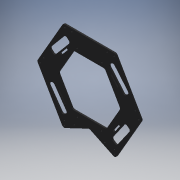
# Autodesk Inventor part: Bottom Plate
Saved by Autodesk Inventor 2017 (Build 210142000, 142)
## iProperties
Created: 2016-10-01
Part Number: Bottom Plate
Material: PVC, Unplasticized
Document SubType Name: Modeling
Designer: James Yelland
Density: 1.29 g/cm^3
Appearance: Smooth - White
Mass: 37.5584 g
Surface Area: 327.952 cm^2
Volume: 29.115 cm^3
Author: James Yelland
Autodesk Inventor part; units mm, degrees
ref_plane "YZ Plane" through (0, 0, 0) normal (1, 0, 0) x (0, 1, 0)
ref_plane "XZ Plane" through (0, 0, 0) normal (0, 1, 0) x (-1, 0, 0)
ref_plane "XY Plane" through (0, 0, 0) normal (0, 0, 1) x (1, 0, 0)
sketch "Sketch1" plane through (0, 0, 0) normal (0, 1, 0) x (-1, 0, 0)
  line L0 (68.7536, -48.1418) -> (56.7085, -65.344)
  line L1 (68.7536, -48.1418) -> (80.7987, -30.9396)
  line L2 (79.8164, -25.3687) -> (75.7207, -22.5008)
  line L3 (70.1498, -23.4831) -> (46.0595, -57.8875)
  line L4 (47.0418, -63.4584) -> (51.1376, -66.3263)
  arc A0 (51.1376, -66.3263) -> (56.7085, -65.344) centre (53.4319, -63.0497) ccw
  arc A1 (46.0595, -57.8875) -> (47.0418, -63.4584) centre (49.3361, -60.1818) ccw
  arc A2 (75.7207, -22.5008) -> (70.1498, -23.4831) centre (73.4264, -25.7774) ccw
  arc A3 (80.7987, -30.9396) -> (79.8164, -25.3687) centre (77.5221, -28.6453) ccw
  line L5 (-68.7536, -48.1418) -> (-80.7987, -30.9396)
  line L6 (-68.7536, -48.1418) -> (-56.7085, -65.344)
  line L7 (-51.1376, -66.3263) -> (-47.0418, -63.4584)
  line L8 (-46.0595, -57.8875) -> (-70.1496, -23.4833)
  line L9 (-75.7207, -22.5008) -> (-79.8164, -25.3687)
  arc A4 (-79.8164, -25.3687) -> (-80.7987, -30.9396) centre (-77.5221, -28.6453) ccw
  arc A5 (-70.1496, -23.4833) -> (-75.7207, -22.5008) centre (-73.4264, -25.7774) ccw
  arc A6 (-47.0418, -63.4584) -> (-46.0595, -57.8875) centre (-49.3361, -60.1818) ccw
  arc A7 (-56.7085, -65.344) -> (-51.1376, -66.3263) centre (-53.4319, -63.0497) ccw
  line L10 (103.5566, -2.5) -> (54.8095, -86.9325)
  line L11 (-54.8095, -86.9325) -> (-103.5566, -2.5)
  line L12 (-103.5566, 2.5) -> (-53.9434, 88.4327)
  line L13 (-49.6132, 90.9327) -> (49.6132, 90.9327)
  line L14 (53.9434, 88.4327) -> (103.5566, 2.5)
  line L15 (2.1497, -66.9563) -> (48.3297, -88.9468)
  line L16 (-2.1497, -66.9563) -> (-48.3297, -88.9468)
  arc A8 (48.3297, -88.9468) -> (54.8095, -86.9325) centre (50.4794, -84.4325) ccw
  arc A9 (2.1497, -66.9563) -> (-2.1497, -66.9563) centre (0, -71.4706) ccw
  arc A10 (-54.8095, -86.9325) -> (-48.3297, -88.9468) centre (-50.4794, -84.4325) ccw
  arc A11 (-103.5566, 2.5) -> (-103.5566, -2.5) centre (-99.2265, 0) ccw
  arc A12 (-49.6132, 90.9327) -> (-53.9434, 88.4327) centre (-49.6132, 85.9327) ccw
  arc A13 (53.9434, 88.4327) -> (49.6132, 90.9327) centre (49.6132, 85.9327) ccw
  arc A14 (103.5566, -2.5) -> (103.5566, 2.5) centre (99.2265, 0) ccw
  circle A15 centre (49.6132, 85.9327) radius 1.6
  circle A16 centre (-49.6132, 85.9327) radius 1.6
  circle A17 centre (-99.2265, 0) radius 1.6
  circle A18 centre (99.2265, 0) radius 1.6
  circle A19 centre (-25, 62.282) radius 1.6
  circle A20 centre (25, 62.282) radius 1.6
  circle A21 centre (24, -57.282) radius 1.6
  circle A22 centre (-24, -57.282) radius 1.6
  line L17 (64.2962, 53.9509) -> (50.7976, 70.0378)
  line L18 (64.2962, 53.9509) -> (77.7947, 37.8639)
  line L19 (77.3017, 32.2286) -> (73.4714, 29.0147)
  line L20 (67.8362, 29.5076) -> (40.839, 61.6816)
  line L21 (41.3321, 67.3169) -> (45.1623, 70.5308)
  arc A23 (50.7976, 70.0378) -> (45.1623, 70.5308) centre (47.7334, 67.4667) ccw
  arc A24 (41.3321, 67.3169) -> (40.839, 61.6816) centre (43.9032, 64.2527) ccw
  arc A25 (67.8362, 29.5076) -> (73.4714, 29.0147) centre (70.9003, 32.0789) ccw
  arc A26 (77.3017, 32.2286) -> (77.7947, 37.8639) centre (74.7305, 35.2928) ccw
  arc A27 (-45.1623, 70.5308) -> (-50.7976, 70.0378) centre (-47.7334, 67.4667) ccw
  line L22 (-45.1623, 70.5308) -> (-41.3321, 67.3169)
  arc A28 (-40.839, 61.6816) -> (-41.3321, 67.3169) centre (-43.9032, 64.2527) ccw
  line L23 (-64.2962, 53.9509) -> (-50.7976, 70.0378)
  line L24 (-40.839, 61.6816) -> (-67.836, 29.5079)
  line L25 (-64.2962, 53.9509) -> (-77.7947, 37.8639)
  arc A29 (-77.7947, 37.8639) -> (-77.3017, 32.2286) centre (-74.7305, 35.2928) ccw
  line L26 (-73.4714, 29.0147) -> (-77.3017, 32.2286)
  arc A30 (-73.4714, 29.0147) -> (-67.836, 29.5079) centre (-70.9003, 32.0789) ccw
  circle A31 centre (50.4794, -84.4325) radius 1.45
  circle A32 centre (50.4794, -76.4325) radius 1.45
  circle A33 centre (-50.4794, -76.4325) radius 1.45
  circle A34 centre (-50.4794, -84.4325) radius 1.45
  circle A35 centre (-30.6147, -73.9104) radius 1.6
  circle A36 centre (30.6147, -73.9104) radius 1.6
  circle A37 centre (35.5991, 85.9437) radius 1.6
  circle A38 centre (-35.5945, 85.9327) radius 1.6
  circle A39 centre (92.2171, 12.1406) radius 1.6
  circle A40 centre (-92.2171, 12.1406) radius 1.6
  arc A41 (31.3397, -49.282) -> (35.6699, -46.782) centre (31.3397, -44.282) ccw
  line L27 (31.3397, -49.282) -> (-31.3397, -49.282)
  arc A42 (-35.6699, -46.782) -> (-31.3397, -49.282) centre (-31.3397, -44.282) ccw
  line L28 (-35.6699, -46.782) -> (-61.2361, -2.5)
  arc A43 (-61.2361, 2.5) -> (-61.2361, -2.5) centre (-56.906, 0) ccw
  line L29 (-61.2361, 2.5) -> (-32.7831, 51.782)
  arc A44 (-28.453, 54.282) -> (-32.7831, 51.782) centre (-28.453, 49.282) ccw
  line L30 (-28.453, 54.282) -> (28.453, 54.282)
  arc A45 (32.7831, 51.782) -> (28.453, 54.282) centre (28.453, 49.282) ccw
  line L31 (32.7831, 51.782) -> (61.2361, 2.5)
  arc A46 (61.2361, -2.5) -> (61.2361, 2.5) centre (56.906, 0) ccw
  line L32 (61.2361, -2.5) -> (35.6699, -46.782)
  line L33 (55.852, -39.108) -> (50.0589, -47.3814)
  line L34 (50.0589, -47.3814) -> (47.4376, -45.546)
  line L35 (47.4376, -45.546) -> (59.0238, -28.9991)
  line L36 (59.0238, -28.9991) -> (61.6451, -30.8345)
  line L37 (61.6451, -30.8345) -> (55.852, -39.108)
  line L38 (43.2875, 49.5071) -> (56.2718, 34.033)
  line L39 (58.7231, 36.0899) -> (52.231, 43.827)
  line L40 (56.2718, 34.033) -> (58.7231, 36.0899)
  line L41 (45.7388, 51.564) -> (43.2875, 49.5071)
  line L42 (52.231, 43.827) -> (45.7388, 51.564)
  line L43 (-61.6451, -30.8345) -> (-55.852, -39.108)
  line L44 (-47.4376, -45.546) -> (-59.0238, -28.9991)
  line L45 (-59.0238, -28.9991) -> (-61.6451, -30.8345)
  line L46 (-55.852, -39.108) -> (-50.0589, -47.3814)
  line L47 (-50.0589, -47.3814) -> (-47.4376, -45.546)
  line L48 (-45.7388, 51.564) -> (-43.2875, 49.5071)
  line L49 (-52.231, 43.827) -> (-45.7388, 51.564)
  line L50 (-58.7231, 36.0899) -> (-52.231, 43.827)
  line L51 (-56.2718, 34.033) -> (-58.7231, 36.0899)
  line L52 (-43.2875, 49.5071) -> (-56.2718, 34.033)
  circle A47 centre (0, 0) radius 6.2089
  point P0 (54.4142, -68.6206)
  point P1 (83.093, -27.663)
  point P2 (72.4441, -20.2065)
  point P3 (43.7652, -61.1641)
  point P4 (-83.093, -27.663)
  point P5 (-54.4142, -68.6206)
  point P6 (-43.7652, -61.1641)
  point P7 (-72.4441, -20.2065)
  point P8 (105, 0)
  point P9 (52.5, -90.9327)
  point P10 (-105, 0)
  point P11 (-52.5, 90.9327)
  point P12 (52.5, 90.9327)
  point P13 (48.2265, 73.102)
  point P14 (80.3658, 34.7998)
  point P15 (70.4073, 26.4435)
  point P16 (38.2679, 64.7458)
  point P17 (-38.2679, 64.7458)
  point P18 (-48.2265, 73.102)
  point P19 (-70.4073, 26.4435)
  point P20 (-80.3658, 34.7998)
  dimension "d11" = 360
  dimension "d30" = 360
  dimension "d90" = 360
  dimension "d136" = 360
  constraints: 106 end point, 58 point on circle, 54 centre point, 45 point on line, 6 coincident
extrude "Extrusion1" add sketch "Sketch1" along normal blind 3 contours L10 A8 L15 A9 L16 A10 L11 A11 L12 A12 L13 A13 L14 A14
body "Solid1"
